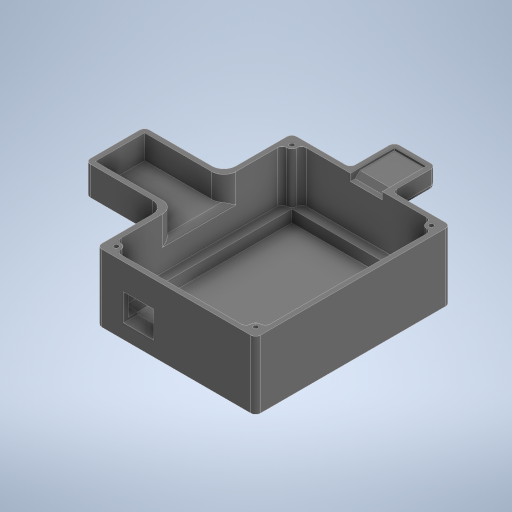
# Autodesk Inventor part: Suporte UNO
Saved by Autodesk Inventor 2023 (Build 270158000, 158)
## iProperties
Created: 2023-06-01
Part Number: Suporte UNO
Material: Genérico
Document SubType Name: Modeling
Designer: Inteli
Density: 1 g/cm^3
Appearance: Cinza
Author: Inteli
Autodesk Inventor part; units mm, degrees
ref_plane "YZ Plane" through (0, 0, 0) normal (1, 0, 0) x (0, 1, 0)
ref_plane "XZ Plane" through (0, 0, 0) normal (0, 1, 0) x (-1, 0, 0)
ref_plane "XY Plane" through (0, 0, 0) normal (0, 0, 1) x (1, 0, 0)
sketch "Esboço1" plane through (0, 0, 0) normal (0, 1, 0) x (-1, 0, 0)
  line L0 (0, 0) -> (65.8, 0)
  line L1 (65.8, 0) -> (65.8, -80.8)
  line L2 (65.8, -80.8) -> (0, -80.8)
  line L3 (0, -80.8) -> (0, 0)
  dimension "d0" = 80.8
  dimension "d1" = 65.8
  constraints: 8 end point, 2 parallel, 1 horizontal, 1 perpendicular
  measures "d0" distance of L0.end L1.end
  measures "d1" distance of L1.end L2.end
extrude "Extrusão1" add sketch "Esboço1" along normal blind 2
sketch "Esboço3" plane through (0, 2, 0) normal (0, 1, 0) x (1, 0, 0)
  line L0 (-65.8, 80.8) -> (-65.8, 0) projected
  line L1 (0, 80.8) -> (-65.8, 80.8) projected
  line L2 (-65.8, 0) -> (0, 0)
  line L3 (0, 0) -> (0, 80.8)
  line L4 (0, 80.8) -> (-65.8, 80.8)
  line L5 (-65.8, 80.8) -> (-65.8, 0)
  line L6 (-6, 6) -> (-59.8, 6)
  line L7 (-59.8, 6) -> (-59.8, 74.8)
  line L8 (-59.8, 74.8) -> (-6, 74.8)
  line L9 (-6, 74.8) -> (-6, 6)
  point P0 (0, 0)
  dimension "d5" = 6
  constraints: 16 end point, 4 parallel, 2 perpendicular, 1 horizontal, 3 other
  measures "d5" distance between parallel lines of L2 L6
extrude "Extrusão2" add sketch "Esboço3" along normal blind 5
sketch "Esboço4" plane through (0, 7, 0) normal (0, 1, 0) x (1, 0, 0)
  line L0 (-65.8, 80.8) -> (-65.8, 0) projected
  line L1 (0, 80.8) -> (-65.8, 80.8) projected
  line L2 (-65.8, 0) -> (0, 0)
  line L3 (0, 0) -> (0, 80.8)
  line L4 (0, 80.8) -> (-65.8, 80.8)
  line L5 (-65.8, 80.8) -> (-65.8, 0)
  line L6 (-2, 2) -> (-63.8, 2)
  line L7 (-63.8, 2) -> (-63.8, 78.8)
  line L8 (-63.8, 78.8) -> (-2, 78.8)
  line L9 (-2, 78.8) -> (-2, 2)
  point P0 (0, 0)
  dimension "d8" = 2
  constraints: 16 end point, 4 parallel, 2 perpendicular, 1 horizontal, 3 other
  measures "d8" distance between parallel lines of L2 L6
extrude "Extrusão3" add sketch "Esboço4" along normal blind 21
sketch "Esboço5" plane through (0, 28, 0) normal (0, 1, 0) x (1, 0, 0)
  line L0 (-63.8, 2) -> (-63.8, 78.8) projected
  line L1 (-6, 6) -> (-59.8, 6) projected
  line L2 (-63.8, 2) -> (-59.8, 2)
  line L3 (-59.8, 2) -> (-59.8, 6)
  line L4 (-59.8, 6) -> (-63.8, 6)
  line L5 (-63.8, 6) -> (-63.8, 2)
  line L6 (-63.8, 78.8) -> (-59.8, 78.8)
  line L7 (-59.8, 78.8) -> (-59.8, 74.8)
  line L8 (-59.8, 74.8) -> (-63.8, 74.8)
  line L9 (-63.8, 74.8) -> (-63.8, 78.8)
  line L10 (-63.8, 2) -> (-2, 2) projected
  line L11 (-2, 2) -> (-6, 2)
  line L12 (-6, 2) -> (-6, 6)
  line L13 (-6, 6) -> (-2, 6)
  line L14 (-2, 6) -> (-2, 2)
  line L15 (-2, 78.8) -> (-2, 2) projected
  line L16 (-2, 78.8) -> (-6, 78.8)
  line L17 (-6, 78.8) -> (-6, 74.8)
  line L18 (-6, 74.8) -> (-2, 74.8)
  line L19 (-2, 74.8) -> (-2, 78.8)
  point P0 (0, 0)
  point P1 (-2, 74.8)
  constraints: 32 end point, 8 parallel, 4 horizontal, 4 perpendicular, 1 point on line
extrude "Extrusão4" add sketch "Esboço5" against normal blind 21 contours L0 L4 L3 L2 | L12 L13 L14 L10 | L0 L6 L7 L8 | L15 L18 L17 L16
sketch "Esboço6" plane through (0, 28, 0) normal (0, 1, 0) x (1, 0, 0)
  circle A0 centre (-61.8, 4) radius 0.95
  line L0 (-59.8, 6) -> (-63.8, 6) projected
  line L1 (-59.8, 2) -> (-59.8, 6) projected
  circle A1 centre (-61.8, 76.8) radius 0.95
  line L2 (-63.8, 74.8) -> (-59.8, 74.8) projected
  line L3 (-59.8, 74.8) -> (-59.8, 78.8) projected
  circle A2 centre (-4, 4) radius 0.95
  line L4 (-6, 6) -> (-6, 2) projected
  line L5 (-2, 6) -> (-6, 6) projected
  circle A3 centre (-4, 76.8) radius 0.95
  line L6 (-6, 78.8) -> (-6, 74.8) projected
  line L7 (-6, 74.8) -> (-2, 74.8) projected
  line L8 (0, 80.8) -> (-65.8, 80.8) projected
  line L9 (0, 0) -> (0, 80.8) projected
  line L10 (-65.8, 0) -> (0, 0) projected
  line L11 (-65.8, 80.8) -> (-65.8, 0) projected
  point P0 (-61.8, 6)
  point P1 (-4, 74.8)
  dimension "d13" = 1.9
  dimension "d16" = 1.9
  dimension "d17" = 2
  dimension "d18" = 2
  dimension "d19" = 1.9
  dimension "d22" = 1.9
  dimension "d71" = 4
  dimension "d72" = 4
  dimension "d73" = 4
  dimension "d74" = 4
  dimension "d75" = 4
  dimension "d76" = 4
  constraints: 4 centre point, 2 midpoint
  measures "d13" diameter of A0
  measures "d16" diameter of A1
  measures "d17" distance from line of L2 A1.centre
  measures "d18" distance from line of L3 A1.centre
  measures "d19" diameter of A2
  measures "d22" diameter of A3
  measures "d71" distance from line of L8 A3.centre
  measures "d72" distance from line of L9 A3.centre
  measures "d73" distance from line of L10 A2.centre
  measures "d74" distance from line of L9 A2.centre
  measures "d75" distance from line of L10 A0.centre
  measures "d76" distance from line of L11 A0.centre
extrude "Extrusão5" cut sketch "Esboço6" against normal blind 7 contours A0 | A1 | A2 | A3
sketch "Esboço7" plane through (-65.8, 0, 0) normal (0, 0, 1) x (1, 0, 0)
  line L0 (11, 17.2) -> (23.5, 17.2)
  line L1 (23.5, 17.2) -> (23.5, 6)
  line L2 (23.5, 6) -> (11, 6)
  line L3 (11, 6) -> (11, 17.2)
  line L4 (0, 0) -> (65.8, 0) projected
  line L5 (0, 0) -> (0, 28) projected
  dimension "d28" = 12.5
  dimension "d29" = 11.2
  dimension "d30" = 6
  dimension "d31" = 11
  constraints: 8 end point, 2 parallel, 1 horizontal, 1 perpendicular
  measures "d28" distance of L1.end L2.end
  measures "d29" distance of L0.end L1.end
  measures "d30" distance between parallel lines of L4 L2
  measures "d31" distance between parallel lines of L3 L5
extrude "Extrusão6" cut sketch "Esboço7" against normal blind 6
sketch "Esboço8" plane through (-65.8, 0, -80.8) normal (-1, 0, 0) x (0, 0, 1)
  line L0 (28.15, 28) -> (52.65, 28)
  line L1 (52.65, 28) -> (52.65, 16)
  line L2 (52.65, 16) -> (28.15, 16)
  line L3 (28.15, 16) -> (28.15, 28)
  line L4 (0, 28) -> (80.8, 28) projected
  line L5 (80.8, 0) -> (80.8, 28) projected
  line L6 (0, 0) -> (0, 28) projected
  dimension "d34" = 24.5
  dimension "d35" = 12
  dimension "d36" = 0
  dimension "d37" = 80.8
  dimension "d38" = 28.15
  constraints: 8 end point, 2 parallel, 1 horizontal, 1 perpendicular
  measures "d34" distance of L1.end L2.end
  measures "d35" distance of L0.end L1.end
  measures "d36" distance between parallel lines of L0 L4
  measures "d37" distance between parallel lines of L5 L6
  measures "d38" distance between parallel lines of L6 L3
extrude "Extrusão7" add sketch "Esboço8" along normal blind 32.9
sketch "Esboço9" plane through (0, 28, 0) normal (0, 1, 0) x (1, 0, 0)
  line L0 (-98.7, 28.15) -> (-98.7, 52.65) projected
  line L1 (-63.8, 6) -> (-63.8, 74.8) projected
  line L2 (-98.7, 28.15) -> (-63.8, 28.15)
  line L3 (-63.8, 28.15) -> (-63.8, 52.65)
  line L4 (-63.8, 52.65) -> (-98.7, 52.65)
  line L5 (-98.7, 52.65) -> (-98.7, 28.15)
  line L6 (-63.8, 30.15) -> (-96.7, 30.15)
  line L7 (-96.7, 30.15) -> (-96.7, 50.65)
  line L8 (-96.7, 50.65) -> (-63.8, 50.65)
  point P0 (0, 0)
  dimension "d41" = 24.5
  dimension "d42" = 2
  constraints: 14 end point, 3 parallel, 3 point on line, 1 horizontal, 1 perpendicular
  measures "d41" distance of L3.end L2.end
  measures "d42" distance between parallel lines of L2 L6
extrude "Extrusão8" cut sketch "Esboço9" against normal blind 10 contours L6 L7 L8 L1
fillet "Arredondamento1" radius 2 6 edges at (-98.7, 22, -28.15) (-98.7, 22, -52.65) (-65.8, 14, 0) (0, 14, 0) (0, 14, -80.8) (-65.8, 14, -80.8)
sketch "Esboço11" plane through (0, 0, 0) normal (0, -1, 0) x (1, 0, 0)
  line L0 (0, -2) -> (0, -78.8) projected
  line L1 (-27.6561, -60.65) -> (-65.6561, -60.65)
  line L2 (-65.6561, -60.65) -> (-65.6561, -68.65)
  line L3 (-65.6561, -68.65) -> (-27.6561, -68.65)
  line L4 (-27.6561, -68.65) -> (-27.6561, -60.65)
  line L5 (-65.6561, -20.15) -> (-27.6561, -20.15)
  line L6 (-27.6561, -20.15) -> (-27.6561, -12.15)
  line L7 (-27.6561, -12.15) -> (-65.6561, -12.15)
  line L8 (-65.6561, -12.15) -> (-65.6561, -20.15)
  line L9 (-27.6561, -64.65) -> (-65.6561, -64.65)
  line L10 (-65.6561, -16.15) -> (-27.6561, -16.15)
  line L11 (-63.8, 0) -> (-2, 0) projected
  line L12 (-2, -80.8) -> (-63.8, -80.8) projected
  point P0 (0, 0)
  point P1 (0, -12.15)
  point P2 (0, -20.15)
  point P3 (0, -68.65)
  dimension "d51" = 38
  dimension "d52" = 8
  dimension "d53" = 8
  dimension "d54" = 4
  dimension "d55" = 4
  dimension "d56" = 48.5
  dimension "d57" = 80.8
  dimension "d58" = 56.5
  dimension "d59" = 12.15
  constraints: 20 end point, 4 midpoint, 4 parallel, 2 horizontal, 2 perpendicular, 2 point on line
  measures "d51" distance of L3.end L2.end
  measures "d52" distance of L2.end L1.end
  measures "d53" distance of L6.end L5.end
  measures "d54" distance between parallel lines of L7 L10
  measures "d55" distance between parallel lines of L9 L3
  measures "d56" distance between parallel lines of L10 L9
  measures "d57" distance between parallel lines of L11 L12
  measures "d58" distance between parallel lines of L7 L3
  measures "d59" distance between parallel lines of L11 L7
extrude "Extrusão10" add sketch "Esboço11" along normal blind 12
sketch "Esboço12" plane through (0, 0, -78.8) normal (1, 0, 0) x (0, 0, -1)
  line L0 (-65.6522, -8) -> (-64.1511, -5.4)
  line L1 (-64.1511, -5.4) -> (-61.1489, -5.4)
  line L2 (-61.1489, -5.4) -> (-59.6478, -8)
  line L3 (-59.6478, -8) -> (-61.1489, -10.6)
  line L4 (-61.1489, -10.6) -> (-64.1511, -10.6)
  line L5 (-64.1511, -10.6) -> (-65.6522, -8)
  line L6 (-17.1522, -8) -> (-15.6511, -5.4)
  line L7 (-15.6511, -5.4) -> (-12.6489, -5.4)
  line L8 (-12.6489, -5.4) -> (-11.1478, -8)
  line L9 (-11.1478, -8) -> (-12.6489, -10.6)
  line L10 (-12.6489, -10.6) -> (-15.6511, -10.6)
  line L11 (-15.6511, -10.6) -> (-17.1522, -8)
  line L12 (-58.65, -12) -> (-66.65, -12) projected
  line L13 (-66.65, 0) -> (-66.65, -12) projected
  line L14 (-18.15, 0) -> (-18.15, -12) projected
  line L15 (-10.15, -12) -> (-18.15, -12) projected
  point P0 (-78.8, 0)
  point P1 (-62.65, -8)
  point P2 (-14.15, -8)
  point P3 (-62.65, -12)
  dimension "d62" = 5.2
  dimension "d63" = 5.2
  dimension "d64" = 4
  dimension "d65" = 4
  dimension "d66" = 4
  dimension "d67" = 4
  constraints: 24 end point, 1 midpoint, 26 other
  measures "d62" distance between parallel lines of L7 L10
  measures "d63" distance between parallel lines of L1 L4
  measures "d64" distance of point (-62.65, -12) point (-62.65, -8)
  measures "d65" distance from line of L13 point (-62.65, -8)
  measures "d66" distance from line of L14 point (-14.15, -8)
  measures "d67" distance from line of L15 point (-14.15, -8)
extrude "Extrusão11" cut sketch "Esboço12" against normal blind 98.7
fillet "Arredondamento2" radius 2 4 edges at (-46.6561, -12, -68.65) (-46.6561, -12, -60.65) (-46.6561, -12, -20.15) (-46.6561, -12, -12.15)
fillet "Arredondamento3" radius 5 3 edges at (-65.8, 22, -28.15) (-65.8, 22, -52.65) (-65.8, 16, -40.4)
fillet "Arredondamento4" radius 5 4 edges at (-46.6561, 0, -12.15) (-46.6561, 0, -20.15) (-46.6561, 0, -68.65) (-46.6561, 0, -60.65)
fillet "Arredondamento5" radius 5 2 edges at (-63.8, 23, -30.15) (-63.8, 23, -50.65)
fillet "Arredondamento6" radius 2 12 edges at (-59.8, 17.5, -2) (-63.8, 17.5, -6) (-59.8, 17.5, -6) (-6, 17.5, -2) (-6, 17.5, -6) (-2, 17.5, -6) (-63.8, 17.5, -74.8) (-59.8, 17.5, -74.8) (-59.8, 17.5, -78.8) (-6, 17.5, -78.8) (-6, 17.5, -74.8) (-2, 17.5, -74.8)
fillet "Arredondamento7" radius 2 1 edges at (-63.8, 18, -40.4)
sketch "Esboço13" plane through (0, 28, 0) normal (0, 1, 0) x (1, 0, 0)
  line L0 (-2, 80.8) -> (-63.8, 80.8) projected
  line L1 (-41.5, 80.8) -> (-24.3, 80.8)
  line L2 (-24.3, 80.8) -> (-24.3, 99)
  line L3 (-24.3, 99) -> (-41.5, 99)
  line L4 (-41.5, 99) -> (-41.5, 80.8)
  line L5 (0, 2) -> (0, 78.8) projected
  line L6 (-65.8, 78.8) -> (-65.8, 57.65) projected
  point P0 (0, 0)
  dimension "d82" = 17.2
  dimension "d83" = 18.2
  dimension "d94" = 65.8
  dimension "d95" = 24.3
  constraints: 8 end point, 2 parallel, 1 horizontal, 1 perpendicular, 1 point on line
  measures "d82" distance of L3.end L2.end
  measures "d83" distance of L2.end L1.end
  measures "d94" distance between parallel lines of L5 L6
  measures "d95" distance between parallel lines of L4 L6
extrude "Extrusão12" add sketch "Esboço13" against normal blind 3
sketch "Esboço14" plane through (0, 28, 0) normal (0, 1, 0) x (1, 0, 0)
  line L0 (-2, 80.8) -> (-63.8, 80.8) projected
  line L1 (-39.5, 80.8) -> (-26.3, 80.8)
  line L2 (-26.3, 80.8) -> (-26.3, 97)
  line L3 (-26.3, 97) -> (-39.5, 97)
  line L4 (-39.5, 97) -> (-39.5, 80.8)
  line L5 (-41.5, 99) -> (-41.5, 80.8) projected
  point P0 (0, 0)
  dimension "d86" = 13.2
  dimension "d87" = 16.2
  dimension "d88" = 2
  constraints: 8 end point, 2 parallel, 1 horizontal, 1 perpendicular, 1 point on line
  measures "d86" distance of L3.end L2.end
  measures "d87" distance of L2.end L1.end
  measures "d88" distance between parallel lines of L5 L4
extrude "Extrusão13" cut sketch "Esboço14" against normal blind 1
sketch "Esboço15" plane through (0, 28, 0) normal (0, 1, 0) x (1, 0, 0)
  line L0 (-26.3, 80.8) -> (-39.5, 80.8) projected
  line L1 (-57.8, 78.8) -> (-8, 78.8) projected
  line L2 (-39.5, 80.8) -> (-26.3, 80.8)
  line L3 (-26.3, 80.8) -> (-26.3, 78.8)
  line L4 (-26.3, 78.8) -> (-39.5, 78.8)
  line L5 (-39.5, 78.8) -> (-39.5, 80.8)
  point P0 (0, 0)
  dimension "d91" = 13.2
  constraints: 8 end point, 2 parallel, 1 horizontal, 1 perpendicular, 1 point on line
  measures "d91" distance of L3.end L4.end
extrude "Extrusão14" cut sketch "Esboço15" against normal blind 3
sketch "Esboço16" plane through (0, 25, 0) normal (0, -1, 0) x (1, 0, 0)
  line L0 (-41.5, -99) -> (-24.3, -99) projected
  line L1 (-24.3, -99) -> (-41.5, -99)
  line L2 (-41.5, -99) -> (-41.5, -80.8)
  line L3 (-41.5, -80.8) -> (-24.3, -80.8)
  line L4 (-24.3, -80.8) -> (-24.3, -99)
  point P0 (0, 0)
  dimension "d96" = 17.2
  dimension "d97" = 18.2
  constraints: 8 end point, 2 parallel, 1 horizontal, 1 perpendicular
  measures "d96" distance of L2.end L3.end
  measures "d97" distance of L1.end L2.end
extrude "Extrusão15" add sketch "Esboço16" along normal blind 5
fillet "Arredondamento8" radius 2 8 edges at (-32.9, 20, -80.8) (-41.5, 24, -80.8) (-24.3, 24, -80.8) (-41.5, 20, -89.9) (-32.9, 20, -99) (-24.3, 20, -89.9) (-24.3, 24, -99) (-41.5, 24, -99)
chamfer "Chanfro1" distance 2 angle 45 1 edges at (-32.9, 27, -80.8)
equation "\"d38\" = -0.5 * d34 + 0.5 * d37"
equation "\"d95\" = -0.5 * d82 + 0.5 * d94"
